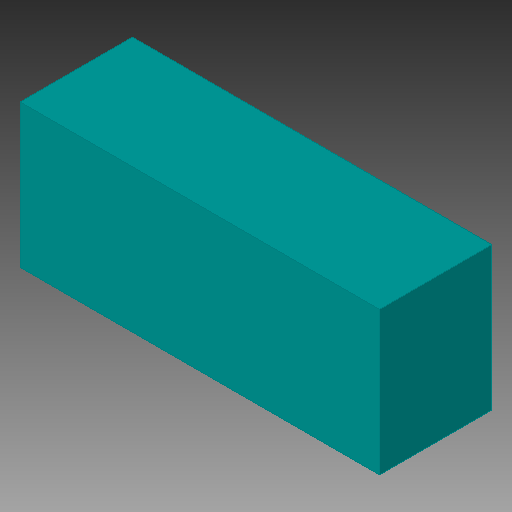
# Autodesk Inventor part: A_3216-18R
Saved by Autodesk Inventor 2018 (Build 220112000, 112)
## iProperties
Created: 2015-11-24
Part Number: A_3216-18R
Material: Generic
Document SubType Name: Modeling
Designer: PhillipD
Density: 1 g/cm^3
Appearance: A_3216-18R, A_3216-18R
Author: PhillipD
Autodesk Inventor part; units mm, degrees
ref_plane "YZ Plane" through (0, 0, 0) normal (1, 0, 0) x (0, 1, 0)
ref_plane "XZ Plane" through (0, 0, 0) normal (0, 1, 0) x (-1, 0, 0)
ref_plane "XY Plane" through (0, 0, 0) normal (0, 0, 1) x (1, 0, 0)
sketch "A_3216-18R, A_3216-18R_14" plane through (0, 0, 0) normal (0, 0, 1) x (1, 0, 0)
  line L0 (-1.6, 0.6508) -> (1.6, 0.6508)
  line L1 (1.6, 0.6508) -> (1.6, -0.625)
  line L2 (1.6, -0.625) -> (-1.6, -0.625)
  line L3 (-1.6, -0.625) -> (-1.6, 0.6508)
  constraints: 8 end point
extrude "Extrusion1" add sketch "A_3216-18R, A_3216-18R_14" along normal blind 1
body "Solid1"
